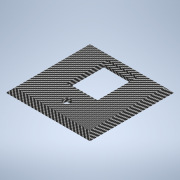
# Autodesk Inventor part: Base Plate
Saved by Autodesk Inventor 2021.1 (Build 251245010, 245A)
## iProperties
Created: 2020-11-23
Part Number: Base Plate
Material: CFRP
Document SubType Name: Modeling
Designer: elizh
Density: 1.43 g/cm^3
Appearance: Carbon Fiber
Author: elizh
Autodesk Inventor part; units mm, degrees
ref_plane "YZ Plane" through (0, 0, 0) normal (1, 0, 0) x (0, 1, 0)
ref_plane "XZ Plane" through (0, 0, 0) normal (0, 1, 0) x (-1, 0, 0)
ref_plane "XY Plane" through (0, 0, 0) normal (0, 0, 1) x (1, 0, 0)
sketch "Sketch1" plane through (0, 0, 0) normal (0, 1, 0) x (-1, 0, 0)
  line L0 (45, 45) -> (-45, 45)
  line L1 (-45, 45) -> (-45, -45)
  line L2 (-45, -45) -> (45, -45)
  line L3 (45, -45) -> (45, 45)
  line L4 (0, 0) -> (55.2623, 0) construction
  line L5 (0, 0) -> (0, -72.148) construction
  dimension "d0" = 90
  constraints: 12 end point, 2 horizontal, 2 parallel, 2 perpendicular, 1 vertical, 2 other
  measures "d0" distance of L2.end L0.start
extrude "Extrusion1" add sketch "Sketch1" along normal blind 5
chamfer "Chamfer2" distance 5 angle 45 4 edges at (-45, 5, 0) (0, 5, -45) (45, 5, 0) (0, 5, 45)
sketch "Sketch5" plane through (0, 5, 0) normal (0, 1, 0) x (1, 0, 0)
  line L0 (0, 0) -> (0, -33.9966) construction
  line L1 (16, -9) -> (-16, -9)
  line L2 (-16, -9) -> (-16, 35)
  line L3 (-16, 35) -> (16, 35)
  line L4 (16, 35) -> (16, -9)
  line L5 (-40, 40) -> (40, 40) construction
  dimension "d13" = 32
  dimension "d14" = 44
  dimension "d15" = 5
  constraints: 10 end point, 2 parallel, 1 horizontal, 1 perpendicular, 1 vertical, 1 other
  measures "d13" distance of L1.start L1.end
  measures "d14" distance of L1.end L2.end
  measures "d15" distance between parallel lines of L5 L3
extrude "Extrusion3" cut sketch "Sketch5" against normal blind 2
sketch "Sketch7" plane through (0, 3, 0) normal (0, 1, 0) x (1, 0, 0)
  line L0 (-16, 35) -> (16, 35) construction
  line L1 (-16, -9) -> (-16, 35) construction
  line L2 (16, -9) -> (-16, -9) construction
  line L3 (16, 35) -> (16, -9) construction
  line L4 (16, -6) -> (-16, -6)
  line L5 (-16, -6) -> (-16, 31)
  line L6 (-16, 31) -> (16, 31)
  line L7 (16, 31) -> (16, -6)
  line L8 (16, 35) -> (16, -9) construction
  line L9 (-16, -9) -> (-16, 35) projected
  dimension "d20" = 3
  dimension "d21" = 4
  constraints: 8 end point, 2 collinear, 2 parallel, 1 horizontal, 1 perpendicular
  measures "d20" distance between parallel lines of L4 L2
  measures "d21" distance between parallel lines of L0 L6
extrude "Extrusion4" cut sketch "Sketch7" against normal through all
sketch "Sketch8" plane through (0, 5, 0) normal (0, 1, 0) x (1, 0, 0)
  circle A0 centre (0, -25) radius 4
  line L0 (0, 0) -> (0, -49.1813) construction
  line L1 (40, -40) -> (-40, -40) construction
  dimension "d24" = 8
  dimension "d25" = 15
  constraints: 2 end point, 1 centre point, 1 point on line, 1 vertical
  measures "d24" diameter of A0
  measures "d25" distance from line of L1 A0.centre
extrude "Extrusion5" cut sketch "Sketch8" against normal through all
sketch "Sketch10" plane through (0, 0, 0) normal (0, -1, 0) x (1, 0, 0)
  circle A0 centre (0, 25) radius 4 construction
  circle A1 centre (0, 25) radius 5
  point P0 (0, 0)
  dimension "d29" = 10
  constraints: 1 centre point, 1 coincident
  measures "d29" diameter of A1
extrude "Extrusion6" cut sketch "Sketch10" against normal blind 4
body "Solid1"
